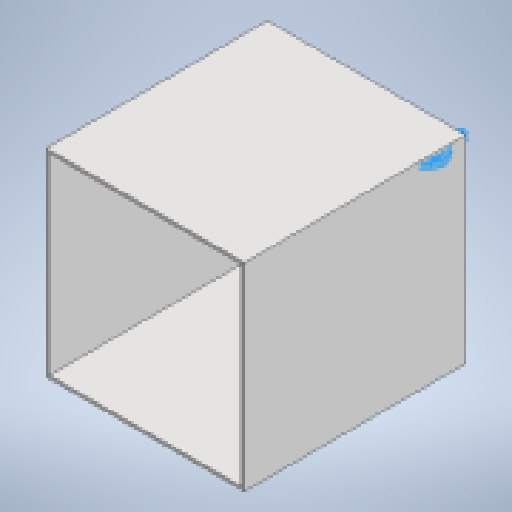
# Autodesk Inventor part: Envolvente
Saved by Autodesk Inventor 2024 (Build 280153000, 153)
## iProperties
Created: 2024-07-16
Part Number: Envolvente
Material: Genérico
Document SubType Name: Modeling
Designer: sergi
Density: 1 g/cm^3
Appearance: Valor por defecto
Author: sergi
Autodesk Inventor part; units mm, degrees
ref_plane "YZ Plane" through (0, 0, 0) normal (1, 0, 0) x (0, 1, 0)
ref_plane "XZ Plane" through (0, 0, 0) normal (0, 1, 0) x (-1, 0, 0)
ref_plane "XY Plane" through (0, 0, 0) normal (0, 0, 1) x (1, 0, 0)
sketch "Boceto1" plane through (0, 0, 0) normal (0, 0, 1) x (1, 0, 0)
  line L0 (-200, -198) -> (-200, 0) projected
  line L1 (-200, -198) -> (-198, -198) projected
  line L2 (-198, 0) -> (-198, -198) projected
  line L3 (-200, 0) -> (-198, 0) projected
  line L4 (-198, 0) -> (0, 0) projected
  line L5 (-198, 0) -> (-198, -2) projected
  line L6 (0, -2) -> (-198, -2) projected
  line L7 (0, 0) -> (0, -2) projected
  line L8 (0, -2) -> (0, -200) projected
  line L9 (0, -2) -> (-2, -2) projected
  line L10 (-2, -200) -> (-2, -2) projected
  line L11 (0, -200) -> (-2, -200) projected
  line L12 (-2, -200) -> (-200, -200) projected
  line L13 (-2, -200) -> (-2, -198) projected
  line L14 (-200, -198) -> (-2, -198) projected
  line L15 (-200, -200) -> (-200, -198) projected
  line L16 (-200, -200) -> (0, -200)
  line L17 (0, -200) -> (0, 0)
  line L18 (0, 0) -> (-200, 0)
  line L19 (-200, 0) -> (-200, -200)
  line L20 (0, 0) -> (0, 3)
  line L21 (0, 3) -> (3, 3)
  line L22 (-200, -200) -> (-203, -200)
  line L23 (-203, -200) -> (-203, -203)
  line L24 (-203, -203) -> (3, -203)
  line L25 (3, -203) -> (3, 3)
  line L26 (3, 3) -> (-203, 3)
  line L27 (-203, 3) -> (-203, -203)
  dimension "espesor" = 3
  dimension "d1" = 3
  dimension "d2" = 3
  dimension "d3" = 3
  constraints: 24 end point, 4 horizontal, 4 parallel, 3 perpendicular, 1 point on line
  measures "espesor" distance of L4.end L20.end
  measures "d1" distance of L20.end L21.end
  measures "d2" distance of L12.end L22.end
  measures "d3" distance of L22.end L23.end
extrude "Extrusión1" add sketch "Boceto1" along normal blind 220 and the other way blind 30 contours L15 L22 L27 L26 L20 L4 L3 L0 | L12 L11 L8 L7 L20 L21 L25 L24 L23 L22
equation "\"d1\" = espesor"
equation "\"d2\" = espesor"
equation "\"d3\" = espesor"
